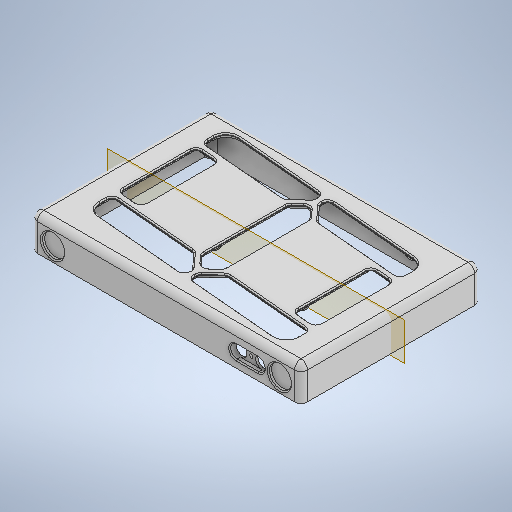
# Autodesk Inventor part: 7Segment
Saved by Autodesk Inventor 2025.2 (Build 292293000, 293)
## iProperties
Created: 2026-02-05
Part Number: 7Segment
Material: Generic
Document SubType Name: Modeling
Designer: Joefi
Density: 1 g/cm^3
Appearance: Default
Author: Joefi
Autodesk Inventor part; units mm, degrees
ref_plane "YZ Plane" through (0, 0, 0) normal (1, 0, 0) x (0, 1, 0)
ref_plane "XZ Plane" through (0, 0, 0) normal (0, 1, 0) x (-1, 0, 0)
ref_plane "XY Plane" through (0, 0, 0) normal (0, 0, 1) x (1, 0, 0)
sketch "Sketch1" plane through (0, 0, 0) normal (0, 1, 0) x (-1, 0, 0)
  line L0 (-119, 83.3333) -> (119, 83.3333)
  line L1 (125, 77.3333) -> (125, -77.3333)
  line L2 (119, -83.3333) -> (-119, -83.3333)
  line L3 (-125, -77.3333) -> (-125, 77.3333)
  line L4 (-125, 83.3333) -> (125, -83.3333) construction
  line L5 (125, 83.3333) -> (-125, -83.3333) construction
  arc A0 (125, 77.3333) -> (119, 83.3333) centre (119, 77.3333) ccw
  arc A1 (119, -83.3333) -> (125, -77.3333) centre (119, -77.3333) ccw
  arc A2 (-125, -77.3333) -> (-119, -83.3333) centre (-119, -77.3333) ccw
  arc A3 (-119, 83.3333) -> (-125, 77.3333) centre (-119, 77.3333) ccw
  line L6 (-125, 83.3333) -> (-119, 83.3333) construction
  line L7 (-125, 83.3333) -> (-125, 77.3333) construction
  point P0 (0, 0)
  dimension "d0" = 250
  dimension "d1" = 166.6667
  dimension "d2" = 6
  constraints: 16 end point, 10 tangent, 8 point on circle, 8 point on line, 4 centre point, 3 equal radius, 2 horizontal, 2 midpoint, 2 parallel, 2 perpendicular
  measures "d0" distance of L4.end L5.end
  measures "d1" distance of L5.start L4.end
  measures "d2" radius of A0
extrude "Extrusion1" add sketch "Sketch1" along normal blind 1.6
sketch "Sketch3" plane through (0, 1.6, 0) normal (0, 1, 0) x (1, 0, 0)
  line L0 (-99.6195, 72.7156) -> (99.6195, 55.2844) construction
  line L1 (99.6195, 55.2844) -> (99.6195, -72.7156) construction
  line L2 (99.6195, -72.7156) -> (-99.6195, -55.2844) construction
  line L3 (-99.6195, -55.2844) -> (-99.6195, 72.7156) construction
  line L4 (0, 64) -> (0, -64) construction
  arc A0 (99.6195, 45.2048) -> (89.5782, 56.1629) centre (88.6195, 45.2048) ccw
  arc A1 (87.6608, -71.6693) -> (99.6195, -60.7112) centre (88.6195, -60.7112) ccw
  arc A2 (-99.6195, -45.2048) -> (-89.5782, -56.1629) centre (-88.6195, -45.2048) ccw
  arc A3 (-87.6608, 71.6693) -> (-99.6195, 60.7112) centre (-88.6195, 60.7112) ccw
  line L5 (-87.6608, 71.6693) -> (-3, 64.2625)
  line L6 (-3, 56.2625) -> (-17.0304, 43.4059)
  line L7 (-17.0304, 43.4059) -> (-99.6195, 50.6315)
  line L8 (-3, 56.2625) -> (-3, 64.2625)
  line L9 (-89.5782, -56.1629) -> (-3, -63.7375)
  line L10 (-3, -63.7375) -> (-3, -55.7375)
  line L11 (-3, -55.7375) -> (-17.0304, -40.426)
  line L12 (-17.0304, -40.426) -> (-99.6195, -33.2004)
  line L13 (-99.6195, -33.2004) -> (-99.6195, -45.2048)
  line L14 (-99.6195, 50.6315) -> (-99.6195, 60.7112)
  line L15 (3, 63.7375) -> (3, 55.7375)
  line L16 (3, 55.7375) -> (17.0304, 40.426)
  line L17 (17.0304, 40.426) -> (99.6195, 33.2004)
  line L18 (89.5782, 56.1629) -> (3, 63.7375)
  line L19 (87.6608, -71.6693) -> (3, -64.2625)
  line L20 (3, -64.2625) -> (3, -56.2625)
  line L21 (3, -56.2625) -> (17.0304, -43.4059)
  line L22 (17.0304, -43.4059) -> (99.6195, -50.6315)
  line L23 (99.6195, 45.2048) -> (99.6195, 33.2004)
  line L24 (99.6195, -60.7112) -> (99.6195, -50.6315)
  line L25 (99.6195, 27.1775) -> (99.6195, -44.6086)
  line L26 (99.6195, -44.6086) -> (77.7032, -42.6912)
  line L27 (77.7032, -42.6912) -> (77.7032, 29.0949)
  line L28 (77.7032, 29.0949) -> (99.6195, 27.1775)
  line L29 (-99.6195, 44.6086) -> (-77.7032, 42.6912)
  line L30 (-77.7032, 42.6912) -> (-77.7032, -29.0949)
  line L31 (-77.7032, -29.0949) -> (-99.6195, -27.1775)
  line L32 (-99.6195, 44.6086) -> (-99.6195, -27.1775)
  line L33 (11, 38.869) -> (11, -40.7938)
  line L34 (11, 38.869) -> (0, 50.8734)
  line L35 (11, -40.7938) -> (0, -50.8734)
  line L36 (0, -50.8734) -> (-11, -38.869)
  line L37 (0, 50.8734) -> (-11, 40.7938)
  line L38 (-11, 40.7938) -> (-11, -38.869)
  point P0 (0, 0)
  point P1 (0, 0)
  point P2 (-3, -59.7375)
  dimension "d16" = 95
  dimension "d17" = 128
  dimension "d20" = 3
  dimension "d21" = 3
  dimension "d24" = 200
  dimension "d25" = 3
  dimension "d27" = 3
  dimension "d29" = 22
  dimension "d31" = 22
  dimension "d32" = 8
  dimension "d34" = 6
  dimension "d35" = 6
  dimension "d36" = 22
  dimension "d37" = 22
  dimension "d38" = 6
  dimension "d39" = 6
  dimension "d43" = 6
  dimension "d44" = 22
  dimension "d46" = 6
  dimension "d49" = 11
  constraints: 78 end point, 22 point on line, 18 tangent, 13 parallel, 8 collinear, 8 point on circle, 8 vertical, 5 equal length, 4 centre point, 4 midpoint, 2 perpendicular, 1 coincident
  measures "d16" angle of L3 L2
  measures "d17" distance of L2.end L0.start
  measures "d20" distance between parallel lines of L4 L10
  measures "d21" distance between parallel lines of L4 L8
  measures "d24" distance of L1.end L2.end
  measures "d25" distance between parallel lines of L4 L15
  measures "d27" distance between parallel lines of L4 L20
  measures "d29" distance between parallel lines of L19 L22
  measures "d31" distance between parallel lines of L0 L17
  measures "d32" distance of L9.end L10.end
  measures "d34" distance between parallel lines of L26 L22
  measures "d35" distance between parallel lines of L17 L28
  measures "d36" distance of L30.end L31.end
  measures "d37" distance of L25.end L26.end
  measures "d38" distance between parallel lines of L12 L31
  measures "d39" distance between parallel lines of L7 L29
  measures "d43" distance between parallel lines of L21 L35
  measures "d44" distance between parallel lines of L33 L38
  measures "d46" distance between parallel lines of L6 L37
  measures "d49" distance between parallel lines of L33 L4
extrude "Extrusion3" cut sketch "Sketch3" against normal blind 30
sketch "Sketch4" plane through (0, 0, 0) normal (0, -1, 0) x (1, 0, 0)
  line L0 (119, -83.3333) -> (-119, -83.3333) projected
  arc A0 (119, -83.3333) -> (125, -77.3333) centre (119, -77.3333) ccw projected
  line L1 (125, 77.3333) -> (125, -77.3333) projected
  arc A1 (125, 77.3333) -> (119, 83.3333) centre (119, 77.3333) ccw projected
  line L2 (-119, 83.3333) -> (119, 83.3333) projected
  arc A2 (-119, 83.3333) -> (-125, 77.3333) centre (-119, 77.3333) ccw projected
  line L3 (-125, -77.3333) -> (-125, 77.3333) projected
  arc A3 (-125, -77.3333) -> (-119, -83.3333) centre (-119, -77.3333) ccw projected
  line L4 (119, 71.3333) -> (119, -71.3333)
  line L5 (113, -77.3333) -> (-113, -77.3333)
  line L6 (-119, -71.3333) -> (-119, 71.3333)
  line L7 (-113, 77.3333) -> (113, 77.3333)
  arc A4 (-119, 83.3333) -> (-125, 77.3333) centre (-119, 77.3333) ccw
  arc A5 (-119, 71.3333) -> (-113, 77.3333) centre (-119, 77.3333) ccw
  arc A6 (-125, -77.3333) -> (-119, -83.3333) centre (-119, -77.3333) ccw
  arc A7 (-113, -77.3333) -> (-119, -71.3333) centre (-119, -77.3333) ccw
  arc A8 (119, -83.3333) -> (125, -77.3333) centre (119, -77.3333) ccw
  arc A9 (119, -71.3333) -> (113, -77.3333) centre (119, -77.3333) ccw
  arc A10 (125, 77.3333) -> (119, 83.3333) centre (119, 77.3333) ccw
  arc A11 (113, 77.3333) -> (119, 71.3333) centre (119, 77.3333) ccw
  point P0 (0, 0)
  dimension "d50" = 6
  constraints: 16 end point, 16 point on circle, 8 centre point
  measures "d50" distance between parallel lines of L2 L7
extrude "Extrusion4" add sketch "Sketch4" along normal blind 30
sketch "Sketch5" plane through (0, 0, 0) normal (0, -1, 0) x (1, 0, 0)
  arc A0 (-99.6195, -60.7112) -> (-87.6608, -71.6693) centre (-88.6195, -60.7112) ccw projected
  line L0 (-99.6195, -60.7112) -> (-99.6195, -50.6315) projected
  line L1 (-99.6195, -50.6315) -> (-17.0304, -43.4059) projected
  line L2 (-17.0304, -43.4059) -> (-3, -56.2625) projected
  line L3 (-3, -56.2625) -> (-3, -64.2625) projected
  line L4 (-3, -64.2625) -> (-87.6608, -71.6693) projected
  line L5 (77.7032, 42.6912) -> (99.6195, 44.6086) projected
  line L6 (99.6195, 44.6086) -> (99.6195, -27.1775) projected
  line L7 (99.6195, -27.1775) -> (77.7032, -29.0949) projected
  line L8 (77.7032, -29.0949) -> (77.7032, 42.6912) projected
  line L9 (-77.7032, 29.0949) -> (-77.7032, -42.6912) projected
  line L10 (-77.7032, -42.6912) -> (-99.6195, -44.6086) projected
  line L11 (-99.6195, -44.6086) -> (-99.6195, 27.1775) projected
  line L12 (-99.6195, 27.1775) -> (-77.7032, 29.0949) projected
  line L13 (-11, 38.869) -> (0, 50.8734) projected
  line L14 (0, 50.8734) -> (11, 40.7938) projected
  line L15 (11, 40.7938) -> (11, -38.869) projected
  line L16 (11, -38.869) -> (0, -50.8734) projected
  line L17 (0, -50.8734) -> (-11, -40.7938) projected
  line L18 (-11, -40.7938) -> (-11, 38.869) projected
  line L19 (99.6195, 60.7112) -> (99.6195, 50.6315) projected
  line L20 (99.6195, 50.6315) -> (17.0304, 43.4059) projected
  line L21 (17.0304, 43.4059) -> (3, 56.2625) projected
  line L22 (3, 56.2625) -> (3, 64.2625) projected
  line L23 (3, 64.2625) -> (87.6608, 71.6693) projected
  arc A1 (99.6195, 60.7112) -> (87.6608, 71.6693) centre (88.6195, 60.7112) ccw projected
  line L24 (-3, 63.7375) -> (-3, 55.7375) projected
  line L25 (-3, 55.7375) -> (-17.0304, 40.426) projected
  line L26 (-17.0304, 40.426) -> (-99.6195, 33.2004) projected
  line L27 (-99.6195, 33.2004) -> (-99.6195, 45.2048) projected
  arc A2 (-89.5782, 56.1629) -> (-99.6195, 45.2048) centre (-88.6195, 45.2048) ccw projected
  line L28 (-89.5782, 56.1629) -> (-3, 63.7375) projected
  line L29 (3, -63.7375) -> (3, -55.7375) projected
  line L30 (3, -55.7375) -> (17.0304, -40.426) projected
  line L31 (17.0304, -40.426) -> (99.6195, -33.2004) projected
  line L32 (99.6195, -33.2004) -> (99.6195, -45.2048) projected
  arc A3 (89.5782, -56.1629) -> (99.6195, -45.2048) centre (88.6195, -45.2048) ccw projected
  line L33 (89.5782, -56.1629) -> (3, -63.7375) projected
  line L34 (16.3281, 41.3368) -> (101.6195, 48.7989)
  line L35 (101.6195, 48.7989) -> (101.6195, 60.7112)
  arc A4 (101.6195, 60.7112) -> (87.4864, 73.6617) centre (88.6195, 60.7112) ccw
  line L36 (87.4864, 73.6617) -> (1, 66.0951)
  line L37 (1, 66.0951) -> (1, 55.3824)
  line L38 (1, 55.3824) -> (16.3281, 41.3368)
  line L39 (101.6195, 46.7912) -> (75.7032, 44.5239)
  line L40 (75.7032, 44.5239) -> (75.7032, -31.2775)
  line L41 (75.7032, -31.2775) -> (101.6195, -29.0101)
  line L42 (101.6195, -29.0101) -> (101.6195, 46.7912)
  line L43 (13, -39.6468) -> (13, 41.6738)
  line L44 (13, 41.6738) -> (-0.1234, 53.6991)
  line L45 (-0.1234, 53.6991) -> (-13, 39.6468)
  line L46 (-13, 39.6468) -> (-13, -41.6738)
  line L47 (-13, -41.6738) -> (0.1234, -53.6991)
  line L48 (0.1234, -53.6991) -> (13, -39.6468)
  line L49 (-16.0813, 38.5014) -> (-1, 54.9598)
  line L50 (-1, 54.9598) -> (-1, 65.9202)
  line L51 (-1, 65.9202) -> (-89.7525, 58.1553)
  arc A5 (-89.7525, 58.1553) -> (-101.6195, 45.2048) centre (-88.6195, 45.2048) ccw
  line L52 (-101.6195, 45.2048) -> (-101.6195, 31.0178)
  line L53 (-101.6195, 31.0178) -> (-16.0813, 38.5014)
  line L54 (-1, -55.3824) -> (-16.3281, -41.3368)
  line L55 (-16.3281, -41.3368) -> (-101.6195, -48.7989)
  line L56 (-101.6195, -48.7989) -> (-101.6195, -60.7112)
  arc A6 (-101.6195, -60.7112) -> (-87.4864, -73.6617) centre (-88.6195, -60.7112) ccw
  line L57 (-87.4864, -73.6617) -> (-1, -66.0951)
  line L58 (-1, -66.0951) -> (-1, -55.3824)
  line L59 (16.0813, -38.5014) -> (1, -54.9598)
  line L60 (1, -54.9598) -> (1, -65.9202)
  line L61 (1, -65.9202) -> (89.7525, -58.1553)
  arc A7 (89.7525, -58.1553) -> (101.6195, -45.2048) centre (88.6195, -45.2048) ccw
  line L62 (101.6195, -45.2048) -> (101.6195, -31.0178)
  line L63 (101.6195, -31.0178) -> (16.0813, -38.5014)
  line L64 (-75.7032, -44.5239) -> (-75.7032, 31.2775)
  line L65 (-75.7032, 31.2775) -> (-101.6195, 29.0101)
  line L66 (-101.6195, 29.0101) -> (-101.6195, -46.7912)
  line L67 (-101.6195, -46.7912) -> (-75.7032, -44.5239)
  line L68 (73.7032, 44.3489) -> (15, 39.213)
  line L69 (15, 39.213) -> (15, -36.5884)
  line L70 (15, -36.5884) -> (73.7032, -31.4525)
  line L71 (73.7032, -31.4525) -> (73.7032, 44.3489)
  line L72 (-15, -39.213) -> (-15, 36.5884)
  line L73 (-15, 36.5884) -> (-73.7032, 31.4525)
  line L74 (-73.7032, 31.4525) -> (-73.7032, -44.3489)
  line L75 (-73.7032, -44.3489) -> (-15, -39.213)
  line L76 (103.6195, 60.7112) -> (103.6195, -45.2048)
  line L77 (-103.6195, 45.2048) -> (-103.6195, -62.0377)
  line L78 (89.9268, -60.1477) -> (-87.3121, -75.6541)
  line L79 (87.3121, 75.6541) -> (-89.9268, 60.1477)
  arc A8 (-89.9268, 60.1477) -> (-103.6195, 45.2048) centre (-88.6195, 45.2048) ccw
  arc A9 (-103.6195, -60.7112) -> (-87.3121, -75.6541) centre (-88.6195, -60.7112) ccw
  arc A10 (89.9268, -60.1477) -> (103.6195, -45.2048) centre (88.6195, -45.2048) ccw
  arc A11 (103.6195, 60.7112) -> (87.3121, 75.6541) centre (88.6195, 60.7112) ccw
  point P0 (0, 0)
  dimension "d53" = 2
  dimension "d54" = 2
  dimension "d55" = 2
  dimension "d56" = 2
  dimension "d57" = 2
  dimension "d58" = 2
  dimension "d59" = 2
  dimension "d60" = 2
  dimension "d61" = 2
  dimension "d62" = 2
  dimension "d63" = 2
  dimension "d64" = 2
  dimension "d65" = 2
  dimension "d66" = 2
  dimension "d67" = 2
  dimension "d68" = 2
  constraints: 92 end point, 16 point on circle, 9 parallel, 8 centre point, 8 tangent, 4 coincident, 1 point on line, 1 vertical, 31 other
  measures "d53" distance between parallel lines of L20 L34
  measures "d54" distance between parallel lines of L5 L39
  measures "d55" distance between parallel lines of L15 L43
  measures "d56" distance between parallel lines of L25 L49
  measures "d57" distance between parallel lines of L2 L54
  measures "d58" distance between parallel lines of L30 L59
  measures "d59" distance between parallel lines of L9 L64
  measures "d60" distance between parallel lines of L34 L68
  measures "d61" distance between parallel lines of L40 L71
  measures "d62" distance between parallel lines of L43 L69
  measures "d63" distance between parallel lines of L63 L70
  measures "d64" distance between parallel lines of L55 L75
  measures "d65" distance between parallel lines of L46 L72
  measures "d66" distance between parallel lines of L53 L73
  measures "d67" distance between parallel lines of L74 L64
  measures "d68" distance between parallel lines of L51 L79
extrude "Extrusion5" add sketch "Sketch5" along normal blind 3 contours L76 A10 L78 A9 L77 A8 L79 A11
fillet "Fillet2" radius 5 30 edges at (-3, 0.8, 63.7375) (-3, 0.8, 55.7375) (-17.0304, 0.8, 40.426) (-99.6195, 0.8, 33.2004) (-99.6195, 0.8, 27.1775) (-77.7032, 0.8, 29.0949) (-77.7032, 0.8, -42.6912) (-99.6195, 0.8, -44.6086) (-99.6195, 0.8, -50.6315) (-17.0304, 0.8, -43.4059) (-3, 0.8, -56.2625) (-3, 0.8, -64.2625) (3, 0.8, -55.7375) (3, 0.8, -63.7375) (17.0304, 0.8, -40.426) (99.6195, 0.8, -33.2004) (99.6195, 0.8, -27.1775) (77.7032, 0.8, -29.0949) (77.7032, 0.8, 42.6912) (99.6195, 0.8, 44.6086) (99.6195, 0.8, 50.6315) (17.0304, 0.8, 43.4059) (3, 0.8, 56.2625) (3, 0.8, 64.2625) (0, 0.8, 50.8734) (11, 0.8, 40.7938) (-11, 0.8, 38.869) (-11, 0.8, -40.7938) (0, 0.8, -50.8734) (11, 0.8, -38.869)
sketch "Sketch6" plane through (0, -30, 0) normal (0, -1, 0) x (1, 0, 0)
  arc A0 (119, -71.3333) -> (113, -77.3333) centre (119, -77.3333) ccw projected
  arc A1 (-113, -77.3333) -> (-119, -71.3333) centre (-119, -77.3333) ccw projected
  arc A2 (-119, 71.3333) -> (-113, 77.3333) centre (-119, 77.3333) ccw projected
  arc A3 (113, 77.3333) -> (119, 71.3333) centre (119, 77.3333) ccw projected
  circle A4 centre (119, -77.3333) radius 1.45
  circle A5 centre (119, 77.3333) radius 1.45
  circle A6 centre (-119, 77.3333) radius 1.45
  circle A7 centre (-119, -77.3333) radius 1.45
  point P0 (0, 0)
  dimension "d72" = 2.9
  dimension "d73" = 2.9
  dimension "d74" = 2.9
  dimension "d75" = 2.9
  constraints: 4 centre point, 4 coincident
  measures "d72" diameter of A4
  measures "d73" diameter of A5
  measures "d74" diameter of A6
  measures "d75" diameter of A7
extrude "Extrusion6" cut sketch "Sketch6" against normal blind 12
chamfer "Chamfer2" distance 1 angle 45 4 edges at (-120.45, -30, -77.3333) (-120.45, -30, 77.3333) (117.55, -30, 77.3333) (117.55, -30, -77.3333)
fillet "Fillet3" radius 6 8 edges at (123.2426, 1.6, -81.576) (0, 1.6, -83.3333) (-123.2426, 1.6, -81.576) (-125, 1.6, 0) (-123.2426, 1.6, 81.576) (0, 1.6, 83.3333) (123.2426, 1.6, 81.576) (125, 1.6, 0)
fillet "Fillet4" [suppressed]
sketch "Sketch7" plane through (-119, -30, 83.3333) normal (0, 0, 1) x (1, 0, 0)
  line L0 (0, 0) -> (0, 25.6) projected
  line L1 (238, 0) -> (238, 25.6) projected
  circle A0 centre (14, 12.8) radius 10.25
  circle A1 centre (224, 12.8) radius 10.25
  line L2 (238, 12.8) -> (0, 12.8) construction
  point P0 (119, 30)
  dimension "d83" = 20.5
  dimension "d84" = 20.5
  dimension "d85" = 14
  dimension "d86" = 14
  constraints: 2 centre point, 2 end point, 2 midpoint, 2 point on line, 1 perpendicular
  measures "d83" diameter of A0
  measures "d84" diameter of A1
  measures "d85" distance from line of L1 A1.centre
  measures "d86" distance of L2.end A0.centre
extrude "Extrusion7" cut sketch "Sketch7" against normal blind 3
ref_plane "Work Plane1" through (-119, -30, 0) normal (0, 0, 1) x (1, 0, 0)
sketch "Sketch8" plane through (-119, -30, 83.3333) normal (0, 0, 1) x (1, 0, 0)
  circle A0 centre (224, 12.8) radius 10.25 projected
  circle A1 centre (14, 12.8) radius 10.25 projected
  arc A2 (204, 6.8) -> (204, 18.8) centre (204, 12.8) ccw
  arc A3 (184, 18.8) -> (184, 6.8) centre (184, 12.8) ccw
  line L0 (184, 6.8) -> (204, 6.8)
  line L1 (204, 18.8) -> (184, 18.8)
  line L2 (224, 12.8) -> (14, 12.8) construction
  point P0 (119, 30)
  dimension "d92" = 12
  dimension "d93" = 12
  dimension "d94" = 20
  dimension "d95" = 20
  constraints: 6 end point, 4 point on circle, 4 tangent, 2 centre point, 2 point on line, 1 horizontal
  measures "d92" diameter of A2
  measures "d93" diameter of A3
  measures "d94" distance of A2.centre A3.centre
  measures "d95" distance of L2.start A2.centre
extrude "Extrusion8" cut sketch "Sketch8" against normal blind 4 contours L0 A3 L1 A2
sketch "Sketch9" plane through (-119, -30, 79.3333) normal (0, 0, 1) x (1, 0, 0)
  line L0 (184, 18.8) -> (204, 18.8) projected
  arc A0 (184, 18.8) -> (184, 6.8) centre (184, 12.8) ccw projected
  line L1 (204, 6.8) -> (184, 6.8) projected
  arc A1 (204, 6.8) -> (204, 18.8) centre (204, 12.8) ccw projected
  arc A2 (184, 18.8) -> (184, 6.8) centre (184, 12.8) ccw projected
  line L2 (194, 18.8) -> (194, 6.8) construction
  circle A3 centre (194, 12.8) radius 1.6
  line L3 (190, 6.8) -> (190, 18.8) construction
  line L4 (198, 18.8) -> (198, 6.8) construction
  circle A4 centre (184, 12.8) radius 6
  circle A5 centre (204, 12.8) radius 6
  point P0 (119, 30)
  dimension "d100" = 3.2
  dimension "d101" = 4
  dimension "d102" = 4
  constraints: 6 end point, 4 point on line, 3 centre point, 3 midpoint, 2 coincident, 2 perpendicular
  measures "d100" diameter of A3
  measures "d101" distance between parallel lines of L2 L4
  measures "d102" distance between parallel lines of L3 L2
extrude "Extrusion9" cut sketch "Sketch9" against normal blind 4 contours A4 A0 | A1 A5 | A3
mirror "Mirror2" about plane through (-119, -30, 0) normal (0, 0, 1) of "Extrusion8", "Extrusion9", "Extrusion7"
chamfer "Chamfer4" distance 1 angle 45 12 edges at (75, -23.2, 83.3333) (59, -17.2, 83.3333) (75, -11.2, 83.3333) (91, -17.2, 83.3333) (94.75, -17.2, 83.3333) (-115.25, -17.2, 83.3333) (94.75, -17.2, -83.3333) (91, -17.2, -83.3333) (75, -11.2, -83.3333) (59, -17.2, -83.3333) (75, -23.2, -83.3333) (-115.25, -17.2, -83.3333)
fillet "Fillet6" radius 1 28 edges at (79.3252, 1.6, -27.3247) (89.0971, 1.6, -28.0981) (98.3059, 1.6, -25.9738) (99.6195, 1.6, 8.2781) (97.9974, 1.6, 42.8385) (88.2255, 1.6, 43.6118) (79.0168, 1.6, 41.4875) (77.7032, 1.6, 7.2356) (10.5766, 1.6, 40.6074) (6.5322, 1.6, 44.8878) (0.0903, 1.6, 48.8043) (-6.5322, 1.6, 43.7448) (-10.66, 1.6, 38.7368) (-11, 1.6, -0.8345) (-10.5766, 1.6, -40.6074) (-6.5322, 1.6, -44.8878) (-0.0903, 1.6, -48.8043) (6.5322, 1.6, -43.7448) (10.66, 1.6, -38.7368) (11, 1.6, 0.8345) (-79.3252, 1.6, 27.3247) (-89.0971, 1.6, 28.0981) (-98.3059, 1.6, 25.9738) (-99.6195, 1.6, -8.2781) (-97.9974, 1.6, -42.8385) (-88.2255, 1.6, -43.6118) (-79.0168, 1.6, -41.4875) (-77.7032, 1.6, -7.2356)
fillet "Fillet7" radius 1 40 edges at (17.1791, 1.6, 43.844) (57.1387, 1.6, 46.915) (98.3059, 1.6, 51.8352) (99.6195, 1.6, 57.9622) (96.051, 1.6, 68.8212) (47.6125, 1.6, 68.1656) (4.3136, 1.6, 63.0588) (3, 1.6, 59.0717) (3.4234, 1.6, 56.4488) (10.0152, 1.6, 49.8342) (-3.34, 1.6, 55.8697) (-3, 1.6, 57.9815) (-4.622, 1.6, 61.9674) (-49.007, 1.6, 59.7124) (-96.7295, 1.6, 52.6363) (-99.6195, 1.6, 41.9309) (-97.9974, 1.6, 34.9705) (-56.5756, 1.6, 36.9662) (-17.1918, 1.6, 40.7531) (-10.0152, 1.6, 48.0818) (-10.0152, 1.6, -49.8342) (-3.4234, 1.6, -56.4488) (-3, 1.6, -59.0717) (-4.3136, 1.6, -63.0588) (-47.6125, 1.6, -68.1656) (-96.051, 1.6, -68.8212) (-99.6195, 1.6, -57.9622) (-98.3059, 1.6, -51.8352) (-57.1387, 1.6, -46.915) (-17.1791, 1.6, -43.844) (3.34, 1.6, -55.8697) (3, 1.6, -57.9815) (4.622, 1.6, -61.9674) (49.007, 1.6, -59.7124) (96.7295, 1.6, -52.6363) (99.6195, 1.6, -41.9309) (97.9974, 1.6, -34.9705) (56.5756, 1.6, -36.9662) (17.1918, 1.6, -40.7531) (10.0152, 1.6, -48.0818)
sketch "Sketch10" plane through (0, 0, 0) normal (0, -1, 0) x (1, 0, 0)
  line L0 (-73.7032, 31.4525) -> (-73.7032, -44.3489) projected
  line L1 (-73.7032, -6.4482) -> (73.7032, 6.4482) construction
  line L2 (73.7032, -31.4525) -> (73.7032, 44.3489) construction
  line L3 (-73.7032, 31.4525) -> (-15, -39.213) construction
  line L4 (15, -36.5884) -> (73.7032, -31.4525) construction
  line L5 (15, -36.5884) -> (73.7032, 44.3489) construction
  circle A0 centre (44.3516, 3.8803) radius 6
  circle A1 centre (-44.3516, -3.8803) radius 6
  point P0 (0, 0)
  dimension "d110" = 12
  dimension "d111" = 12
  constraints: 6 end point, 4 midpoint, 2 centre point
  measures "d110" diameter of A0
  measures "d111" diameter of A1
extrude "Extrusion10" add sketch "Sketch10" along normal up to surface (30 mm away)
sketch "Sketch11" plane through (44.3516, -30, 3.8803) normal (0, -1, 0) x (1, 0, 0)
  circle A0 centre (0, 0) radius 6 projected
  circle A1 centre (0, 0) radius 1.45
  circle A2 centre (-88.7032, -7.7605) radius 6 projected
  circle A3 centre (-88.7032, -7.7605) radius 1.45
  point P0 (-44.3516, -3.8803)
  dimension "d114" = 2.9
  dimension "d115" = 2.9
  constraints: 2 centre point, 2 coincident
  measures "d114" diameter of A1
  measures "d115" diameter of A3
extrude "Extrusion11" cut sketch "Sketch11" against normal blind 12 contours A1 | A3
chamfer "Chamfer5" distance 1 angle 45 2 edges at (42.9016, -30, 3.8803) (-45.8016, -30, -3.8803)
chamfer "Chamfer6" distance 3 angle 45 2 edges at (38.3516, 0, 3.8803) (-50.3516, 0, -3.8803)
equation "\"d1\" = 0.666667 * d0"
equation "\"d21\" = d20"
equation "\"d25\" = d20"
equation "\"d27\" = d20"
equation "\"d31\" = d29"
body "Solid1"
